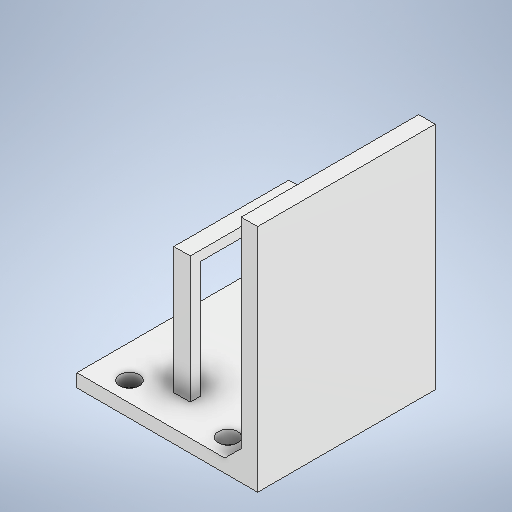
# Autodesk Inventor part: obudowa_łoż_pion_1
Saved by Autodesk Inventor 2025 (Build 290162000, 162)
## iProperties
Created: 2024-04-14
Part Number: obudowa_łoż_pion_1
Material: Tworzywo sztuczne ABS
Document SubType Name: Modeling
Designer: user
Density: 1.06 g/cm^3
Appearance: Gładki — biały
Mass: 31.718 g
Surface Area: 145.422 cm^2
Volume: 29.9226 cm^3
Author: user
Autodesk Inventor part; units mm, degrees
ref_plane "YZ Plane" through (0, 0, 0) normal (1, 0, 0) x (0, 1, 0)
ref_plane "XZ Plane" through (0, 0, 0) normal (0, 1, 0) x (-1, 0, 0)
ref_plane "XY Plane" through (0, 0, 0) normal (0, 0, 1) x (1, 0, 0)
sketch "Szkic1" plane through (0, 0, 0) normal (0, 1, 0) x (-1, 0, 0)
  line L0 (25, 27) -> (-25, 27)
  line L1 (-25, 27) -> (-25, -27)
  line L2 (-25, -27) -> (25, -27)
  line L3 (25, -27) -> (25, 27)
  line L4 (-25, 27) -> (25, -27) construction
  circle A0 centre (15, 21) radius 3
  line L5 (25, 0) -> (-25, 0)
  line L6 (0, 27) -> (0, -27)
  circle A1 centre (15, -21) radius 3
  circle A2 centre (-15, 21) radius 3
  circle A3 centre (-15, -21) radius 3
  line L7 (-25, 27) -> (-30, 27)
  line L8 (-30, 27) -> (-30, -27)
  line L9 (-30, -27) -> (-25, -27)
  line L10 (-25, -27) -> (-25, 27)
  line L11 (0, -14.5) -> (5, -14.5)
  line L12 (5, -14.5) -> (5, -17.5)
  line L13 (5, -17.5) -> (0, -17.5)
  line L14 (0, -17.5) -> (0, -14.5)
  line L15 (0, -14.5) -> (-5, -14.5)
  line L16 (-5, -14.5) -> (-5, -17.5)
  line L17 (-5, -17.5) -> (0, -17.5)
  line L18 (0, 14.5) -> (5, 14.5)
  line L19 (5, 14.5) -> (5, 17.5)
  line L20 (5, 17.5) -> (0, 17.5)
  line L21 (-5, 14.5) -> (-5, 17.5)
  line L22 (-5, 17.5) -> (0, 17.5)
  line L23 (0, 14.5) -> (-5, 14.5)
  line L24 (5, 14.5) -> (5, -14.5)
  line L25 (-5, 14.5) -> (-5, -14.5)
  point P0 (0, 0)
  point P1 (-27.5, 27)
  point P2 (-25, -27)
  point P3 (0, -17.5)
  point P4 (0, 17.5)
  dimension "d0" = 50
  dimension "d5" = 10
  dimension "d7" = 6
  dimension "d8" = 6
  dimension "d9" = 5
  dimension "d10" = 54
  dimension "d12" = 54
  dimension "d21" = 5
  dimension "d22" = 3
  dimension "d26" = 14.5
  dimension "d27" = 50
  dimension "d28" = 36.688
  constraints: 52 end point, 11 symmetric about line, 6 midpoint, 6 parallel, 4 centre point, 3 horizontal, 3 perpendicular, 1 collinear, 1 point on line, 3 other
  measures "d0" distance of L2.end L1.end
  measures "d5" distance from line of A0.centre L3
  measures "d7" distance from line of A0.centre L0
  measures "d8" diameter of A0
  measures "d9" distance between parallel lines of L1 L8
  measures "d10" distance from line of point (-27.5, 27) L9
  measures "d12" distance between parallel lines of L2 L0
  measures "d21" distance of L12.end L13.end
  measures "d22" distance of L11.end L12.end
  measures "d26" distance between parallel lines of L5 L15
  measures "d27" distance from line of point (-25, -27) L3
  measures "d28" distance from line of point (-25, -27) L4
extrude "Wyciągnięcie proste1" add sketch "Szkic1" along normal blind 4 contours L3 L5 L24 L19 L20 L6 L0 | L6 L22 L21 L25 L5 L1 L0 | L3 L2 L6 L13 L12 L24 L5 | L20 L19 L18 L6 | L6 L23 L21 L22 | L24 L11 L6 L5 | L5 L6 L18 L24 | L5 L25 L16 L17 L6 L2 L1 | L6 L5 L25 L23 | L6 L15 L25 L5 | L12 L13 L6 L11 | L17 L16 L15 L6
extrude "Wyciągnięcie proste2" add sketch "Szkic1" along normal blind 70 contours L1 L9 L8 L7
sketch "Szkic3" plane through (-25, 0, 27) normal (0, 0, 1) x (1, 0, 0)
  line L0 (50, 4) -> (50, 70) projected
  line L1 (50, 9) -> (45, 4)
  line L2 (0, 4) -> (50, 4) projected
  line L3 (50, 9) -> (57.0711, 9) construction
  point P0 (25, 0)
  dimension "d17" = 135
  dimension "d18" = 5
  constraints: 4 end point, 2 point on line, 1 equal length, 1 horizontal
  measures "d17" angle of L1 L3
  measures "d18" horizontal distance of L1.start L1.end
extrude "Wyciągnięcie proste3" add sketch "Szkic3" against normal blind 54
extrude "Wyciągnięcie proste4" add sketch "Szkic1" along normal blind 42.5 contours L20 L19 L18 L6 | L12 L13 L6 L11
extrude "Wyciągnięcie proste5" add sketch "Szkic1" along normal blind 42.5 contours L24 L11 L6 L5 | L5 L6 L18 L24
extrude "Wyciągnięcie proste6" cut sketch "Szkic1" along normal blind 39.5 contours L24 L11 L6 L5 | L5 L6 L18 L24
extrude "Wyciągnięcie proste7" add sketch "Szkic1" along normal blind 4 contours L24 L11 L6 L5 | L5 L6 L18 L24
